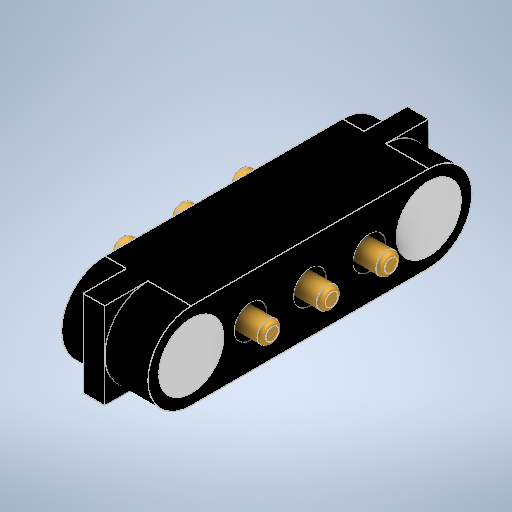
# Autodesk Inventor part: 3_pin_no_ear_male
Saved by Autodesk Inventor 2025.1 (Build 291241000, 241)
## iProperties
Created: 2025-05-04
Part Number: 3_pin_no_ear_male
Material: Generic
Document SubType Name: Modeling
Designer: santiago
Density: 1 g/cm^3
Appearance: Anodized - Black
Author: santiago
Autodesk Inventor part; units mm, degrees
ref_plane "YZ Plane" through (0, 0, 0) normal (1, 0, 0) x (0, 1, 0)
ref_plane "XZ Plane" through (0, 0, 0) normal (0, 1, 0) x (-1, 0, 0)
ref_plane "XY Plane" through (0, 0, 0) normal (0, 0, 1) x (1, 0, 0)
sketch "Sketch1" plane through (0, 0, 0) normal (0, 1, 0) x (-1, 0, 0)
  line L0 (-2, 7.5) -> (2, 7.5)
  line L1 (2, 7.5) -> (2, -7.5)
  line L2 (2, -7.5) -> (-2, -7.5)
  line L3 (-2, -7.5) -> (-2, 7.5)
  line L4 (-2, 7.5) -> (2, -7.5) construction
  line L5 (2, 7.5) -> (-2, -7.5) construction
  point P0 (0, 0)
  dimension "d0" = 4
  dimension "d1" = 15
  constraints: 12 end point, 2 midpoint, 2 parallel, 1 horizontal, 1 perpendicular
  measures "d0" distance of L1.end L2.end
  measures "d1" distance of L0.end L1.end
extrude "Extrusion1" add sketch "Sketch1" along normal blind 4
sketch "Sketch2" plane through (2, 0, 7.5) normal (1, 0, 0) x (0, 0, -1)
  line L0 (0, 0) -> (0, 4) projected
  line L1 (0, 2) -> (15, 2) construction
  line L2 (15, 0) -> (15, 4) projected
  line L3 (2, 0) -> (13, 0)
  line L4 (13, 4) -> (2, 4)
  arc A0 (2, 4) -> (2, 0) centre (2, 2) ccw
  arc A1 (13, 0) -> (13, 4) centre (13, 2) ccw
  line L5 (0, 4) -> (15, 4) projected
  line L6 (0, 0) -> (15, 0) projected
  point P0 (7.5, 0)
  point P1 (7.5, 2)
  point P2 (15, 2)
  constraints: 8 end point, 6 point on circle, 4 tangent, 3 midpoint, 2 centre point, 2 point on line, 1 parallel
extrude "Extrusion2" cut sketch "Sketch2" against normal blind 2 contours L0 A0 L6 | L0 L5 A0 | A1 L2 L6 | L5 L2 A1
sketch "Sketch3" plane through (-2, 0, -7.5) normal (-1, 0, 0) x (0, 0, 1)
  arc A0 (2, 4) -> (0, 2) centre (2, 2) ccw projected
  line L0 (0, 0) -> (0, 4) projected
  line L1 (0, 4) -> (15, 4) projected
  arc A1 (0, 2) -> (2, 0) centre (2, 2) ccw projected
  arc A2 (2, 4) -> (2, 0) centre (2, 2) ccw projected
  line L2 (13, 4) -> (2, 4) projected
  arc A3 (13, 0) -> (13, 4) centre (13, 2) ccw projected
  line L3 (13, 0) -> (2, 0) projected
  line L4 (15, 0) -> (15, 4) projected
  line L5 (0, 0) -> (15, 0) projected
  point P0 (7.5, 0)
  point P1 (15, 2)
extrude "Extrusion3" cut sketch "Sketch3" against normal blind 1 contours A0 L0 L1 | A1 L5 L0 | L1 L4 A3 | L4 L5 A3
sketch "Sketch4" plane through (-2, 0, -5.5) normal (-1, 0, 0) x (0, 0, 1)
  arc A0 (0, 4) -> (-2, 2) centre (0, 2) ccw projected
  circle A1 centre (0, 2) radius 1.5
  arc A2 (13, 2) -> (11, 4) centre (11, 2) ccw projected
  circle A3 centre (11, 2) radius 1.5
  point P0 (5.5, 0)
  dimension "d8" = 3
  dimension "d9" = 3
  constraints: 2 centre point, 2 coincident
  measures "d8" diameter of A1
  measures "d9" diameter of A3
mark "Mark1"
sketch "Sketch5" plane through (-2, 0, -5.5) normal (-1, 0, 0) x (0, 0, 1)
  circle A0 centre (2.75, 2) radius 1
  circle A1 centre (0, 2) radius 1.5 projected
  circle A2 centre (11, 2) radius 1.5 projected
  line L0 (0, 4) -> (11, 4) projected
  circle A3 centre (5.5, 2) radius 1
  circle A4 centre (8.25, 2) radius 1
  point P0 (5.5, 0)
  dimension "d10" = 2
  dimension "d11" = 2.75
  dimension "d12" = 11
  dimension "d15" = 2.75
  constraints: 3 centre point, 1 horizontal, 4 other
  measures "d10" diameter of A0
  measures "d11" distance of A1.centre A0.centre
  measures "d12" distance of A2.centre A1.centre
  measures "d15" distance of A0.centre A3.centre
mark "Mark2"
sketch "Sketch6" plane through (-2, 2, -2.75) normal (-1, 0, 0) x (0, 0, 1)
  circle A0 centre (0, 0) radius 1 projected
  circle A1 centre (0, 0) radius 0.5
  circle A2 centre (2.75, 0) radius 1 projected
  circle A3 centre (2.75, 0) radius 0.5
  circle A4 centre (5.5, 0) radius 1 projected
  circle A5 centre (5.5, 0) radius 0.5
  point P0 (2.75, -2)
  dimension "d20" = 1
  dimension "d21" = 1
  dimension "d31" = 1
  constraints: 3 centre point, 3 coincident
  measures "d20" diameter of A1
  measures "d21" diameter of A3
  measures "d31" diameter of A5
extrude "Extrusion4" add sketch "Sketch6" along normal blind 2 contours A1 | A3 | A5
sketch "Sketch7" plane through (2, 0, 5.5) normal (1, 0, 0) x (0, 0, -1)
  circle A0 centre (0, 2) radius 1.5 projected
  circle A1 centre (11, 2) radius 1.5 projected
  point P0 (5.5, 0)
mark "Mark3"
sketch "Sketch8" plane through (2, 0, 5.5) normal (1, 0, 0) x (0, 0, -1)
  circle A0 centre (8.25, 2) radius 1 projected
  circle A1 centre (5.5, 2) radius 1 projected
  circle A2 centre (5.5, 2) radius 0.75
  circle A3 centre (8.25, 2) radius 0.75
  circle A4 centre (2.75, 2) radius 1 projected
  circle A5 centre (2.75, 2) radius 0.75
  point P0 (5.5, 0)
  dimension "d24" = 1.5
  dimension "d25" = 1.5
  dimension "d32" = 1.5
  constraints: 3 centre point, 3 coincident
  measures "d24" diameter of A2
  measures "d25" diameter of A3
  measures "d32" diameter of A5
extrude "Extrusion5" cut sketch "Sketch8" against normal blind 1 contours A2 | A3 | A5
sketch "Sketch9" plane through (1, 2, 0) normal (1, 0, 0) x (0, 0, -1)
  circle A0 centre (2.75, 0) radius 0.5 projected
  circle A1 centre (0, 0) radius 0.5 projected
  circle A2 centre (-2.75, 0) radius 0.5 projected
  point P0 (0, -2)
extrude "Extrusion6" add sketch "Sketch9" along normal blind 2
fillet "Fillet1" radius 0.2 6 edges at (3, 2, 0.5) (3, 2, -2.25) (-4, 2, -3.25) (-4, 2, -0.5) (3, 2, 3.25) (-4, 2, 2.25)
equation "\"d9\" = d8"
equation "\"d11\" = 0.25 * d12"
equation "\"d15\" = d11"
equation "\"d21\" = d20"
equation "\"d31\" = d21"
equation "\"d25\" = d24"
equation "\"d32\" = d24"
body "Solid1"
